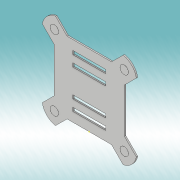
# Autodesk Inventor part: Superior_Base
Saved by Autodesk Inventor 2019 (Build 230136000, 136)
## iProperties
Created: 2019-01-30
Part Number: Superior_Base
Material: Generic
Document SubType Name: Modeling
Designer: USUARIO
Density: 1 g/cm^3
Appearance: Default
Title: Superior_Base
Author: USUARIO
Autodesk Inventor part; units mm, degrees
ref_plane "YZ Plane" through (0, 0, 0) normal (1, 0, 0) x (0, 1, 0)
ref_plane "XZ Plane" through (0, 0, 0) normal (0, 1, 0) x (-1, 0, 0)
ref_plane "XY Plane" through (0, 0, 0) normal (0, 0, 1) x (1, 0, 0)
sketch "Sketch1" plane through (0, 0, 0) normal (0, 0, 1) x (1, 0, 0)
  line L0 (0, 0) -> (-47.5, 0)
  line L1 (-47.5, 0) -> (-72.2487, -24.7487)
  line L2 (-100.4666, 3.6019) -> (-75, 29.0685)
  line L3 (-75, 29.0685) -> (-75, 76.5685)
  line L4 (0, -71.4752) -> (0, 224.6123) projected
  arc A0 (-100.4666, 3.6019) -> (-72.2487, -24.7487) centre (-66, 9.6889) ccw
  line L5 (-75, 76.5685) -> (0, 76.5685)
  line L6 (0, 153.1371) -> (-47.5, 153.1371)
  line L7 (-47.5, 153.1371) -> (-72.2487, 177.8858)
  line L8 (-100.4666, 149.5352) -> (-75, 124.0685)
  line L9 (-75, 124.0685) -> (-75, 76.5685)
  arc A1 (-72.2487, 177.8858) -> (-100.4666, 149.5352) centre (-66, 143.4481) ccw
  line L10 (0, 0) -> (47.5, 0)
  line L11 (47.5, 0) -> (72.2487, -24.7487)
  line L12 (100.4666, 3.6019) -> (75, 29.0685)
  line L13 (75, 29.0685) -> (75, 76.5685)
  arc A2 (72.2487, -24.7487) -> (100.4666, 3.6019) centre (66, 9.6889) ccw
  line L14 (75, 124.0685) -> (75, 76.5685)
  line L15 (100.4666, 149.5352) -> (75, 124.0685)
  arc A3 (100.4666, 149.5352) -> (72.2487, 177.8858) centre (66, 143.4481) ccw
  line L16 (47.5, 153.1371) -> (72.2487, 177.8858)
  line L17 (0, 153.1371) -> (47.5, 153.1371)
  line L18 (-100.4666, 3.6019) -> (-72.2487, -24.7487)
  line L19 (-75, 29.0685) -> (-47.5, 0)
  circle A4 centre (-74.6902, 1.0941) radius 9
  circle A5 centre (-74.6902, 152.043) radius 9
  circle A6 centre (74.6902, 1.0941) radius 9
  circle A7 centre (74.6902, 152.043) radius 9
  dimension "d0" = 135
  dimension "d1" = 47.5
  dimension "d2" = 35
  dimension "d3" = 40
  dimension "d4" = 75
  dimension "d5" = 35
  dimension "d6" = 66
  dimension "d11" = 20
  dimension "d12" = 38
  dimension "d13" = 18
  constraints: 38 end point, 20 symmetric about line, 8 centre point, 8 point on circle, 2 perpendicular, 1 horizontal, 1 midpoint, 1 parallel, 1 vertical, 6 other
  measures "d0" angle of L1 L0
  measures "d1" distance of L0.start L0.end
  measures "d2" distance of L0.end L1.end
  measures "d3" distance between parallel lines of L1 L2
  measures "d4" distance between parallel lines of L4 L3
  measures "d5" radius of A0
  measures "d6" distance from line of L4 A0.centre
  measures "d11" distance from line of L2 A4.centre
  measures "d12" diameter of A4.centre L19
  measures "d13" diameter of A4
extrude "Extrusion1" add sketch "Sketch1" along normal blind 1.5 and the other way blind 1.5 contours L0 L19 L3 L5 L4 | L4 L17 L16 A3 L15 L14 L13 L12 A2 L11 L10 | L1 L18 L2 L19 | L5 L9 L8 A1 L7 L6 L4 | A0 L18 | A4 | A5 | A6 | A7
extrude "Extrusion2" add sketch "Sketch1" along normal mid plane 3.2 contours A4 | A5 | A6 | A7
sketch "Sketch2" plane through (0, 0, 1.5) normal (0, 0, 1) x (1, 0, 0)
  point P0 (0, 0)
sketch "Sketch3" plane through (0, 0, 1.5) normal (0, 0, 1) x (1, 0, 0)
  line L0 (0, 20) -> (-35, 20)
  line L1 (-35, 20) -> (-35, 28)
  line L2 (-35, 28) -> (0, 28)
  line L3 (0, 43) -> (-35, 43)
  line L4 (-35, 43) -> (-35, 51)
  line L5 (-35, 51) -> (0, 51)
  line L6 (0, 0) -> (0, 150)
  line L7 (-75, 124.0685) -> (-75, 29.0685) projected
  line L8 (-75, 76.5685) -> (75, 76.5685)
  line L9 (75, 124.0685) -> (75, 29.0685) projected
  line L10 (0, 133.1371) -> (-35, 133.1371)
  line L11 (-35, 133.1371) -> (-35, 125.1371)
  line L12 (-35, 125.1371) -> (0, 125.1371)
  line L13 (0, 110.1371) -> (-35, 110.1371)
  line L14 (-35, 110.1371) -> (-35, 102.1371)
  line L15 (-35, 102.1371) -> (0, 102.1371)
  line L16 (0, 20) -> (35, 20)
  line L17 (35, 20) -> (35, 28)
  line L18 (35, 28) -> (0, 28)
  line L19 (0, 43) -> (35, 43)
  line L20 (35, 43) -> (35, 51)
  line L21 (35, 51) -> (0, 51)
  line L22 (35, 102.1371) -> (0, 102.1371)
  line L23 (0, 110.1371) -> (35, 110.1371)
  line L24 (35, 110.1371) -> (35, 102.1371)
  line L25 (35, 125.1371) -> (0, 125.1371)
  line L26 (35, 133.1371) -> (35, 125.1371)
  line L27 (0, 133.1371) -> (35, 133.1371)
  dimension "d21" = 35
  dimension "d22" = 8
  dimension "d23" = 150
  dimension "d24" = 15
  dimension "d25" = 20
  constraints: 52 end point, 16 symmetric about line, 4 equal length, 4 perpendicular, 2 horizontal, 2 midpoint, 2 point on line, 1 vertical
  measures "d21" distance of L4.end L5.end
  measures "d22" distance of L3.end L4.end
  measures "d23" distance of L6.start L6.end
  measures "d24" distance between parallel lines of L2 L3
  measures "d25" distance of point (0, 0) L0.start
extrude "Extrusion3" cut sketch "Sketch3" against normal blind 10
body "Solid1"
